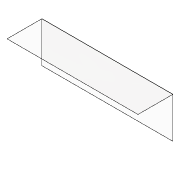
# Autodesk Inventor part: フルクロス
Saved by Autodesk Inventor 2019 (Build 230136000, 136)
## iProperties
Created: 2019-08-16
Part Number: フルクロス
Material: ポリカーボネート、クリア
Document SubType Name: Modeling
Designer: tanjihayato
Density: 1.2 g/cm^3
Appearance: ポリカーボネート - クリア
Author: tanjihayato
Autodesk Inventor part; units mm, degrees
ref_plane "YZ Plane" through (0, 0, 0) normal (1, 0, 0) x (0, 1, 0)
ref_plane "XZ Plane" through (0, 0, 0) normal (0, 1, 0) x (-1, 0, 0)
ref_plane "XY Plane" through (0, 0, 0) normal (0, 0, 1) x (1, 0, 0)
sketch "スケッチ1" plane through (0, 0, 0) normal (0, 0, 1) x (1, 0, 0)
  line L0 (0, 0) -> (450, 0)
  line L1 (450, 0) -> (450, -140)
  line L2 (450, -140) -> (0, -140)
  line L3 (0, -140) -> (0, 0)
  line L4 (0, -0.5) -> (450, -0.5)
  dimension "d0" = 450
  dimension "d1" = 140
  dimension "d2" = 0.5
  constraints: 10 end point, 2 horizontal, 2 parallel, 2 point on line, 1 perpendicular
  measures "d0" distance of L1.end L2.end
  measures "d1" distance of L2.end L0.start
  measures "d2" distance between parallel lines of L0 L4
extrude "押し出し1" add sketch "スケッチ1" along normal blind 0.5 contours L4 L1 L2 L3
extrude "押し出し2" add sketch "スケッチ1" along normal blind 120 contours L0 L1 L4 L3
